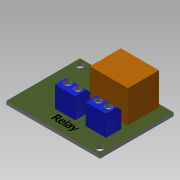
# Autodesk Inventor part: Driver Kipas
Saved by Autodesk Inventor 2015 SP1 (Build 190203100, 203)
## iProperties
Created: 2015-01-28
Part Number: Driver Kipas
Material: Generic
Document SubType Name: Modeling
Designer: Rafi Kurnia Putra
Density: 1 g/cm^3
Appearance: Default
Author: Rafi Kurnia Putra
Autodesk Inventor part; units mm, degrees
ref_plane "YZ Plane" through (0, 0, 0) normal (1, 0, 0) x (0, 1, 0)
ref_plane "XZ Plane" through (0, 0, 0) normal (0, 1, 0) x (-1, 0, 0)
ref_plane "XY Plane" through (0, 0, 0) normal (0, 0, 1) x (1, 0, 0)
sketch "Sketch1" plane through (0, 0, 0) normal (0, 1, 0) x (-1, 0, 0)
  line L0 (23.125, 18.205) -> (-23.125, 18.205)
  line L1 (-23.125, 18.205) -> (-23.125, -18.205)
  line L2 (-23.125, -18.205) -> (23.125, -18.205)
  line L3 (23.125, -18.205) -> (23.125, 18.205)
  line L4 (23.125, 18.205) -> (-23.125, -18.205) construction
  circle A0 centre (20.125, -15.205) radius 1.75
  circle A1 centre (-20.125, 15.205) radius 1.75
  line L5 (23.125, -18.205) -> (-23.125, 18.205) construction
  line L6 (1.475, -16.705) -> (-17.315, -16.705)
  line L7 (-17.315, -16.705) -> (-17.315, -1.385)
  line L8 (-17.315, -1.385) -> (1.475, -1.385)
  line L9 (1.475, -1.385) -> (1.475, -16.705)
  line L10 (1.475, -16.705) -> (-17.315, -1.385) construction
  line L11 (1.475, -1.385) -> (-17.315, -16.705) construction
  circle A2 centre (17.125, 9.445) radius 0.5
  circle A3 centre (17.125, 6.905) radius 0.5
  circle A4 centre (17.125, 4.365) radius 0.5
  circle A5 centre (6.8029, -14.4063) radius 2.5
  circle A6 centre (-9.7762, 5.6314) radius 1.75
  circle A7 centre (-14.7762, 5.6314) radius 1.75
  line L12 (-7.2762, 1.8814) -> (-17.2762, 1.8814)
  line L13 (-17.2762, 1.8814) -> (-17.2762, 9.3814)
  line L14 (-17.2762, 9.3814) -> (-7.2762, 9.3814)
  line L15 (-7.2762, 9.3814) -> (-7.2762, 1.8814)
  line L16 (-7.2762, 1.8814) -> (-17.2762, 9.3814) construction
  line L17 (-17.2762, 1.8814) -> (-7.2762, 9.3814) construction
  circle A8 centre (5.3096, 5.6314) radius 1.75
  circle A9 centre (0.3096, 5.6314) radius 1.75
  line L18 (7.8096, 1.9748) -> (-2.1904, 1.9748)
  line L19 (-2.1904, 1.9748) -> (-2.1904, 9.4748)
  line L20 (-2.1904, 9.4748) -> (7.8096, 9.4748)
  line L21 (7.8096, 9.4748) -> (7.8096, 1.9748)
  line L22 (7.8096, 1.9748) -> (-2.1904, 9.4748) construction
  line L23 (-2.1904, 1.9748) -> (7.8096, 9.4748) construction
  point P0 (0, 0)
  point P1 (0, 0)
  point P2 (0, 0)
  point P3 (-17.2167, 8.2868)
  point P4 (-12.2762, 5.6314)
  point P5 (2.8096, 5.7248)
  dimension "d0" = 46.25
  dimension "d1" = 36.41
  dimension "d5" = 3
  dimension "d6" = 3
  dimension "d7" = 3.5
  dimension "d8" = 3
  dimension "d9" = 3
  dimension "d10" = 18.79
  dimension "d11" = 15.32
  dimension "d12" = 24.2439
  dimension "d13" = 24.2439
  dimension "d14" = 5.81
  dimension "d15" = 1.5
  dimension "d16" = 1
  dimension "d17" = 8.76
  dimension "d18" = 6
  dimension "d19" = 1
  dimension "d20" = 1
  dimension "d21" = 2.54
  dimension "d22" = 2.54
  dimension "d23" = 5
  dimension "d25" = 3.5
  dimension "d26" = 3.5
  dimension "d28" = 5
  dimension "d29" = 10
  dimension "d30" = 7.5
  dimension "d31" = 3.5
  dimension "d32" = 3.5
  dimension "d33" = 5
  dimension "d34" = 2.5
  dimension "d35" = 10
  dimension "d36" = 7.5
  constraints: 48 end point, 10 centre point, 8 parallel, 7 midpoint, 4 horizontal, 4 perpendicular, 1 coincident, 1 horizontal alignment
  measures "d0" distance of L2.end L1.end
  measures "d1" distance of L1.end L0.end
  measures "d5" distance from line of A0.centre L3
  measures "d6" distance from line of A0.centre L2
  measures "d7" diameter of A1
  measures "d8" distance from line of A1.centre L1
  measures "d9" distance from line of A1.centre L0
  measures "d10" distance of L7.end L8.end
  measures "d11" distance of L6.end L7.end
  measures "d12" distance of L6.start L7.end
  measures "d13" distance of L8.end L6.end
  measures "d14" distance between parallel lines of L7 L1
  measures "d15" distance between parallel lines of L6 L2
  measures "d16" diameter of A2
  measures "d17" distance from line of L0 A2.centre
  measures "d18" distance from line of A2.centre L3
  measures "d19" diameter of A3
  measures "d20" diameter of A4
  measures "d21" distance of A3.centre A2.centre
  measures "d22" distance of A4.centre A3.centre
  measures "d23" diameter of A5
  measures "d25" diameter of A6
  measures "d26" diameter of A7
  measures "d28" distance of A7.centre A6.centre
  measures "d29" distance of L13.end L15.start
  measures "d30" distance of L12.end L13.end
  measures "d31" diameter of A8
  measures "d32" diameter of A9
  measures "d33" distance of A8.centre A9.centre
  measures "d34" horizontal distance of A9.centre point (2.81, 5.725)
  measures "d35" distance of L19.end L20.end
  measures "d36" distance of L18.end L19.end
extrude "Extrusion1" add sketch "Sketch1" along normal blind 1.6 contours L3 L2 L1 L0
extrude "Extrusion2" add sketch "Sketch1" along normal blind 17.44 contours L6 L7 L8 L9
extrude "Extrusion3" add sketch "Sketch1" along normal blind 10.15 contours A5
extrude "Extrusion4" add sketch "Sketch1" along normal blind 11.88 contours L12 L13 L14 L15 | L18 L19 L20 L21
chamfer "Chamfer1" distance 2 angle 45 2 edges at (-2.8096, 11.88, 1.9748) (12.2762, 11.88, 1.8814)
extrude "Extrusion5" add sketch "Sketch1" along normal blind 10 contours A6 | A7 | A8 | A9
sketch "Sketch2" plane through (0, 1.6, 0) normal (0, 1, 0) x (1, 0, 0)
  line L0 (-4.8976, -10.9925) -> (20.6377, -10.9925) construction
  line L1 (20.6377, -10.9925) -> (20.6377, -15.4823) construction
  line L2 (20.6377, -15.4823) -> (-4.8976, -15.4823) construction
  line L3 (-4.8976, -15.4823) -> (-4.8976, -10.9925) construction
  point P0 (0, 0)
  constraints: 2 other
sketch "Sketch3" plane through (0, 1.6, 0) normal (0, 1, 0) x (1, 0, 0)
  line L0 (-22.0426, 6.9482) -> (-2.0211, 6.9482) construction
  line L1 (-2.0211, 6.9482) -> (-2.0211, 3.1958) construction
  line L2 (-2.0211, 3.1958) -> (-22.0426, 3.1958) construction
  line L3 (-22.0426, 3.1958) -> (-22.0426, 6.9482) construction
  line L4 (-20.3295, 5.4223) -> (-20.3522, 5.4223)
  spline S0 degree 2 poles (-20.3522, 5.4223) (-20.4032, 5.4365) (-20.5138, 5.4421) (-20.5904, 5.4421) knots 0 0 0 1 2 2 2
  spline S1 degree 2 poles (-20.5904, 5.4421) (-20.7691, 5.4421) (-21.1208, 5.2861) (-21.2796, 5.133) knots 0 0 0 1 2 2 2
  line L5 (-21.2796, 5.133) -> (-21.2796, 3.2695)
  line L6 (-21.2796, 3.2695) -> (-21.7221, 3.2695)
  line L7 (-21.7221, 3.2695) -> (-21.7221, 5.8959)
  line L8 (-21.7221, 5.8959) -> (-21.2796, 5.8959)
  line L9 (-21.2796, 5.8959) -> (-21.2796, 5.5045)
  spline S2 degree 2 poles (-21.2796, 5.5045) (-21.0386, 5.7201) (-20.6783, 5.8959) (-20.5082, 5.8959) knots 0 0 0 1 2 2 2
  spline S3 degree 2 poles (-20.5082, 5.8959) (-20.4401, 5.8959) (-20.372, 5.8903) (-20.3295, 5.8818) knots 0 0 0 1 2 2 2
  line L10 (-20.3295, 5.8818) -> (-20.3295, 5.4223)
  spline S4 degree 2 poles (-18.5228, 3.5475) (-18.5766, 3.5078) (-18.7582, 3.366) (-18.8433, 3.3234) knots 0 0 0 1 2 2 2
  spline S5 degree 2 poles (-18.8433, 3.3234) (-18.9595, 3.261) (-19.1779, 3.1958) (-19.3765, 3.1958) knots 0 0 0 1 2 2 2
  spline S6 degree 2 poles (-19.3765, 3.1958) (-19.5381, 3.1958) (-19.8303, 3.3177) (-19.9409, 3.4284) knots 0 0 0 1 2 2 2
  spline S7 degree 2 poles (-19.9409, 3.4284) (-20.0458, 3.5361) (-20.1735, 3.8538) (-20.1735, 4.0297) knots 0 0 0 1 2 2 2
  spline S8 degree 2 poles (-20.1735, 4.0297) (-20.1735, 4.3019) (-19.9437, 4.6877) (-19.6941, 4.7983) knots 0 0 0 1 2 2 2
  spline S9 degree 2 poles (-19.6941, 4.7983) (-19.4729, 4.9004) (-18.8716, 4.977) (-18.5228, 4.9968) knots 0 0 0 1 2 2 2
  line L11 (-18.5228, 4.9968) -> (-18.5228, 5.0819)
  spline S10 degree 2 poles (-18.5228, 5.0819) (-18.5228, 5.2351) (-18.6164, 5.4251) (-18.7014, 5.479) knots 0 0 0 1 2 2 2
  spline S11 degree 2 poles (-18.7014, 5.479) (-18.7865, 5.5329) (-19.0305, 5.5669) (-19.1609, 5.5669) knots 0 0 0 1 2 2 2
  spline S12 degree 2 poles (-19.1609, 5.5669) (-19.3141, 5.5669) (-19.7282, 5.4762) (-19.9352, 5.3882) knots 0 0 0 1 2 2 2
  line L12 (-19.9352, 5.3882) -> (-19.9608, 5.3882)
  line L13 (-19.9608, 5.3882) -> (-19.9608, 5.8392)
  spline S13 degree 2 poles (-19.9608, 5.8392) (-19.8388, 5.8733) (-19.3822, 5.9583) (-19.1581, 5.9583) knots 0 0 0 1 2 2 2
  spline S14 degree 2 poles (-19.1581, 5.9583) (-18.8858, 5.9583) (-18.5142, 5.8733) (-18.3668, 5.7626) knots 0 0 0 1 2 2 2
  spline S15 degree 2 poles (-18.3668, 5.7626) (-18.2221, 5.6549) (-18.0803, 5.3117) (-18.0803, 5.0649) knots 0 0 0 1 2 2 2
  line L14 (-18.0803, 5.0649) -> (-18.0803, 3.2695)
  line L15 (-18.0803, 3.2695) -> (-18.5228, 3.2695)
  line L16 (-18.5228, 3.2695) -> (-18.5228, 3.5475)
  line L17 (-18.5228, 3.9162) -> (-18.5228, 4.6451)
  spline S16 degree 2 poles (-18.5228, 4.6451) (-18.6816, 4.631) (-19.1609, 4.5827) (-19.3112, 4.5374) knots 0 0 0 1 2 2 2
  spline S17 degree 2 poles (-19.3112, 4.5374) (-19.4871, 4.4835) (-19.7168, 4.2594) (-19.7168, 4.0609) knots 0 0 0 1 2 2 2
  spline S18 degree 2 poles (-19.7168, 4.0609) (-19.7168, 3.834) (-19.4616, 3.6042) (-19.2176, 3.6042) knots 0 0 0 1 2 2 2
  spline S19 degree 2 poles (-19.2176, 3.6042) (-19.0106, 3.6042) (-18.6702, 3.7829) (-18.5228, 3.9162) knots 0 0 0 1 2 2 2
  line L18 (-16.0779, 6.5001) -> (-16.1005, 6.5001)
  spline S20 degree 2 poles (-16.1005, 6.5001) (-16.1601, 6.5228) (-16.3813, 6.5625) (-16.4693, 6.5625) knots 0 0 0 1 2 2 2
  spline S21 degree 2 poles (-16.4693, 6.5625) (-16.7472, 6.5625) (-16.9855, 6.3129) (-16.9855, 5.9839) knots 0 0 0 1 2 2 2
  line L19 (-16.9855, 5.9839) -> (-16.9855, 5.8959)
  line L20 (-16.9855, 5.8959) -> (-16.2537, 5.8959)
  line L21 (-16.2537, 5.8959) -> (-16.2537, 5.5301)
  line L22 (-16.2537, 5.5301) -> (-16.9713, 5.5301)
  line L23 (-16.9713, 5.5301) -> (-16.9713, 3.2695)
  line L24 (-16.9713, 3.2695) -> (-17.4138, 3.2695)
  line L25 (-17.4138, 3.2695) -> (-17.4138, 5.5301)
  line L26 (-17.4138, 5.5301) -> (-17.7116, 5.5301)
  line L27 (-17.7116, 5.5301) -> (-17.7116, 5.8959)
  line L28 (-17.7116, 5.8959) -> (-17.4138, 5.8959)
  line L29 (-17.4138, 5.8959) -> (-17.4138, 5.9839)
  spline S22 degree 2 poles (-17.4138, 5.9839) (-17.4138, 6.4547) (-16.9571, 6.9482) (-16.5317, 6.9482) knots 0 0 0 1 2 2 2
  spline S23 degree 2 poles (-16.5317, 6.9482) (-16.4097, 6.9482) (-16.1743, 6.9227) (-16.0779, 6.9057) knots 0 0 0 1 2 2 2
  line L30 (-16.0779, 6.9057) -> (-16.0779, 6.5001)
  line L31 (-15.4766, 3.2695) -> (-15.919, 3.2695)
  line L32 (-15.919, 3.2695) -> (-15.919, 5.8959)
  line L33 (-15.919, 5.8959) -> (-15.4766, 5.8959)
  line L34 (-15.4766, 5.8959) -> (-15.4766, 3.2695)
  line L35 (-15.4454, 6.3327) -> (-15.9474, 6.3327)
  line L36 (-15.9474, 6.3327) -> (-15.9474, 6.7922)
  line L37 (-15.9474, 6.7922) -> (-15.4454, 6.7922)
  line L38 (-15.4454, 6.7922) -> (-15.4454, 6.3327)
  line L39 (-12.6516, 3.2695) -> (-13.233, 3.2695)
  line L40 (-13.233, 3.2695) -> (-14.2087, 4.5374)
  line L41 (-14.2087, 4.5374) -> (-14.3846, 4.3672)
  line L42 (-14.3846, 4.3672) -> (-14.3846, 3.2695)
  line L43 (-14.3846, 3.2695) -> (-14.827, 3.2695)
  line L44 (-14.827, 3.2695) -> (-14.827, 6.9255)
  line L45 (-14.827, 6.9255) -> (-14.3846, 6.9255)
  line L46 (-14.3846, 6.9255) -> (-14.3846, 4.7869)
  line L47 (-14.3846, 4.7869) -> (-13.3465, 5.8959)
  line L48 (-13.3465, 5.8959) -> (-12.7963, 5.8959)
  line L49 (-12.7963, 5.8959) -> (-13.874, 4.7983)
  line L50 (-13.874, 4.7983) -> (-12.6516, 3.2695)
  line L51 (-10.3882, 3.2695) -> (-10.8307, 3.2695)
  line L52 (-10.8307, 3.2695) -> (-10.8307, 3.5588)
  spline S24 degree 2 poles (-10.8307, 3.5588) (-11.0349, 3.3801) (-11.4008, 3.1958) (-11.6277, 3.1958) knots 0 0 0 1 2 2 2
  spline S25 degree 2 poles (-11.6277, 3.1958) (-11.7979, 3.1958) (-12.1014, 3.3092) (-12.212, 3.4312) knots 0 0 0 1 2 2 2
  spline S26 degree 2 poles (-12.212, 3.4312) (-12.3254, 3.5532) (-12.4502, 3.9247) (-12.4502, 4.1913) knots 0 0 0 1 2 2 2
  line L53 (-12.4502, 4.1913) -> (-12.4502, 5.8959)
  line L54 (-12.4502, 5.8959) -> (-12.0078, 5.8959)
  line L55 (-12.0078, 5.8959) -> (-12.0078, 4.3984)
  spline S27 degree 2 poles (-12.0078, 4.3984) (-12.0078, 4.1885) (-11.9766, 3.9134) (-11.9227, 3.8113) knots 0 0 0 1 2 2 2
  spline S28 degree 2 poles (-11.9227, 3.8113) (-11.8688, 3.7092) (-11.6844, 3.6156) (-11.5114, 3.6156) knots 0 0 0 1 2 2 2
  spline S29 degree 2 poles (-11.5114, 3.6156) (-11.3497, 3.6156) (-10.9839, 3.7999) (-10.8307, 3.9332) knots 0 0 0 1 2 2 2
  line L56 (-10.8307, 3.9332) -> (-10.8307, 5.8959)
  line L57 (-10.8307, 5.8959) -> (-10.3882, 5.8959)
  line L58 (-10.3882, 5.8959) -> (-10.3882, 3.2695)
  line L59 (-8.3546, 5.4223) -> (-8.3773, 5.4223)
  spline S30 degree 2 poles (-8.3773, 5.4223) (-8.4283, 5.4365) (-8.539, 5.4421) (-8.6155, 5.4421) knots 0 0 0 1 2 2 2
  spline S31 degree 2 poles (-8.6155, 5.4421) (-8.7942, 5.4421) (-9.1459, 5.2861) (-9.3048, 5.133) knots 0 0 0 1 2 2 2
  line L60 (-9.3048, 5.133) -> (-9.3048, 3.2695)
  line L61 (-9.3048, 3.2695) -> (-9.7472, 3.2695)
  line L62 (-9.7472, 3.2695) -> (-9.7472, 5.8959)
  line L63 (-9.7472, 5.8959) -> (-9.3048, 5.8959)
  line L64 (-9.3048, 5.8959) -> (-9.3048, 5.5045)
  spline S32 degree 2 poles (-9.3048, 5.5045) (-9.0637, 5.7201) (-8.7035, 5.8959) (-8.5333, 5.8959) knots 0 0 0 1 2 2 2
  spline S33 degree 2 poles (-8.5333, 5.8959) (-8.4652, 5.8959) (-8.3971, 5.8903) (-8.3546, 5.8818) knots 0 0 0 1 2 2 2
  line L65 (-8.3546, 5.8818) -> (-8.3546, 5.4223)
  line L66 (-5.9494, 3.2695) -> (-6.3919, 3.2695)
  line L67 (-6.3919, 3.2695) -> (-6.3919, 4.7671)
  spline S34 degree 2 poles (-6.3919, 4.7671) (-6.3919, 4.9486) (-6.4259, 5.2606) (-6.477, 5.3542) knots 0 0 0 1 2 2 2
  spline S35 degree 2 poles (-6.477, 5.3542) (-6.5309, 5.4535) (-6.7237, 5.5499) (-6.8882, 5.5499) knots 0 0 0 1 2 2 2
  spline S36 degree 2 poles (-6.8882, 5.5499) (-7.0527, 5.5499) (-7.4016, 5.3741) (-7.5689, 5.2322) knots 0 0 0 1 2 2 2
  line L68 (-7.5689, 5.2322) -> (-7.5689, 3.2695)
  line L69 (-7.5689, 3.2695) -> (-8.0114, 3.2695)
  line L70 (-8.0114, 3.2695) -> (-8.0114, 5.8959)
  line L71 (-8.0114, 5.8959) -> (-7.5689, 5.8959)
  line L72 (-7.5689, 5.8959) -> (-7.5689, 5.6038)
  spline S37 degree 2 poles (-7.5689, 5.6038) (-7.3704, 5.7825) (-6.9875, 5.9697) (-6.7719, 5.9697) knots 0 0 0 1 2 2 2
  spline S38 degree 2 poles (-6.7719, 5.9697) (-6.3862, 5.9697) (-5.9494, 5.4592) (-5.9494, 4.9741) knots 0 0 0 1 2 2 2
  line L73 (-5.9494, 4.9741) -> (-5.9494, 3.2695)
  line L74 (-4.8773, 3.2695) -> (-5.3198, 3.2695)
  line L75 (-5.3198, 3.2695) -> (-5.3198, 5.8959)
  line L76 (-5.3198, 5.8959) -> (-4.8773, 5.8959)
  line L77 (-4.8773, 5.8959) -> (-4.8773, 3.2695)
  line L78 (-4.8461, 6.3327) -> (-5.3481, 6.3327)
  line L79 (-5.3481, 6.3327) -> (-5.3481, 6.7922)
  line L80 (-5.3481, 6.7922) -> (-4.8461, 6.7922)
  line L81 (-4.8461, 6.7922) -> (-4.8461, 6.3327)
  spline S39 degree 2 poles (-2.7642, 3.5475) (-2.8181, 3.5078) (-2.9997, 3.366) (-3.0847, 3.3234) knots 0 0 0 1 2 2 2
  spline S40 degree 2 poles (-3.0847, 3.3234) (-3.201, 3.261) (-3.4194, 3.1958) (-3.618, 3.1958) knots 0 0 0 1 2 2 2
  spline S41 degree 2 poles (-3.618, 3.1958) (-3.7796, 3.1958) (-4.0718, 3.3177) (-4.1824, 3.4284) knots 0 0 0 1 2 2 2
  spline S42 degree 2 poles (-4.1824, 3.4284) (-4.2873, 3.5361) (-4.415, 3.8538) (-4.415, 4.0297) knots 0 0 0 1 2 2 2
  spline S43 degree 2 poles (-4.415, 4.0297) (-4.415, 4.3019) (-4.1852, 4.6877) (-3.9356, 4.7983) knots 0 0 0 1 2 2 2
  spline S44 degree 2 poles (-3.9356, 4.7983) (-3.7144, 4.9004) (-3.1131, 4.977) (-2.7642, 4.9968) knots 0 0 0 1 2 2 2
  line L82 (-2.7642, 4.9968) -> (-2.7642, 5.0819)
  spline S45 degree 2 poles (-2.7642, 5.0819) (-2.7642, 5.2351) (-2.8578, 5.4251) (-2.9429, 5.479) knots 0 0 0 1 2 2 2
  spline S46 degree 2 poles (-2.9429, 5.479) (-3.028, 5.5329) (-3.2719, 5.5669) (-3.4024, 5.5669) knots 0 0 0 1 2 2 2
  spline S47 degree 2 poles (-3.4024, 5.5669) (-3.5556, 5.5669) (-3.9697, 5.4762) (-4.1767, 5.3882) knots 0 0 0 1 2 2 2
  line L83 (-4.1767, 5.3882) -> (-4.2023, 5.3882)
  line L84 (-4.2023, 5.3882) -> (-4.2023, 5.8392)
  spline S48 degree 2 poles (-4.2023, 5.8392) (-4.0803, 5.8733) (-3.6236, 5.9583) (-3.3996, 5.9583) knots 0 0 0 1 2 2 2
  spline S49 degree 2 poles (-3.3996, 5.9583) (-3.1273, 5.9583) (-2.7557, 5.8733) (-2.6082, 5.7626) knots 0 0 0 1 2 2 2
  spline S50 degree 2 poles (-2.6082, 5.7626) (-2.4636, 5.6549) (-2.3218, 5.3117) (-2.3218, 5.0649) knots 0 0 0 1 2 2 2
  line L85 (-2.3218, 5.0649) -> (-2.3218, 3.2695)
  line L86 (-2.3218, 3.2695) -> (-2.7642, 3.2695)
  line L87 (-2.7642, 3.2695) -> (-2.7642, 3.5475)
  line L88 (-2.7642, 3.9162) -> (-2.7642, 4.6451)
  spline S51 degree 2 poles (-2.7642, 4.6451) (-2.9231, 4.631) (-3.4024, 4.5827) (-3.5527, 4.5374) knots 0 0 0 1 2 2 2
  spline S52 degree 2 poles (-3.5527, 4.5374) (-3.7286, 4.4835) (-3.9583, 4.2594) (-3.9583, 4.0609) knots 0 0 0 1 2 2 2
  spline S53 degree 2 poles (-3.9583, 4.0609) (-3.9583, 3.834) (-3.7031, 3.6042) (-3.4591, 3.6042) knots 0 0 0 1 2 2 2
  spline S54 degree 2 poles (-3.4591, 3.6042) (-3.2521, 3.6042) (-2.9117, 3.7829) (-2.7642, 3.9162) knots 0 0 0 1 2 2 2
  point P0 (0, 0)
  constraints: 2 other
extrude "Extrusion6" cut sketch "Sketch3" against normal blind 10
body "Solid1"
